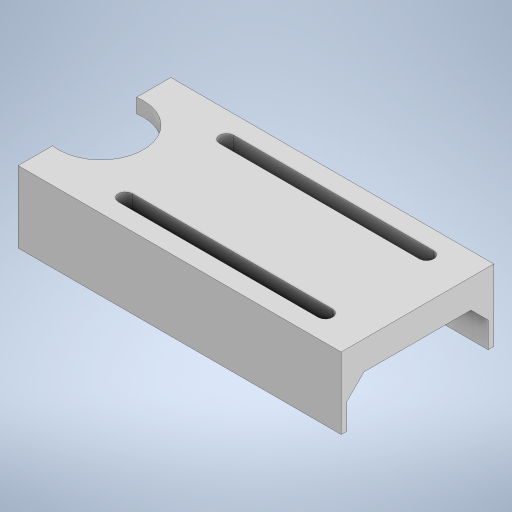
# Autodesk Inventor part: klapa
Saved by Autodesk Inventor 2024.3 (Build 283343000, 343)
## iProperties
Created: 2024-08-09
Part Number: klapa
Material: Ogólny
Document SubType Name: Modeling
Designer: User
Density: 1 g/cm^3
Appearance: Domyślna
Author: User
Autodesk Inventor part; units mm, degrees
ref_plane "YZ Plane" through (0, 0, 0) normal (1, 0, 0) x (0, 1, 0)
ref_plane "XZ Plane" through (0, 0, 0) normal (0, 1, 0) x (-1, 0, 0)
ref_plane "XY Plane" through (0, 0, 0) normal (0, 0, 1) x (1, 0, 0)
sketch "Szkic1" plane through (0, 0, 0) normal (0, 1, 0) x (-1, 0, 0)
  line L0 (0, 0) -> (0, -49.4)
  line L1 (0, 0) -> (108, 0)
  line L2 (0, 0) -> (108.995, 0)
  line L3 (108.995, 0) -> (108.995, -49.4)
  line L4 (108.995, -49.4) -> (0, -49.4)
  line L5 (0, -49.4) -> (0, 0)
  line L6 (0, 0) -> (0, 2)
  line L7 (0, 2) -> (-2, 2)
  line L8 (108.995, -49.4) -> (110.995, -49.4)
  line L9 (110.995, -49.4) -> (110.995, -51.4)
  line L10 (110.995, -51.4) -> (-2, -51.4)
  line L11 (-2, -51.4) -> (-2, 2)
  line L12 (-2, 2) -> (110.995, 2)
  line L13 (110.995, 2) -> (110.995, -51.4)
  line L14 (110.995, 2) -> (100.995, 2)
  line L15 (100.995, 2) -> (100.995, 0)
  line L16 (110.995, -51.4) -> (100.995, -51.4)
  line L17 (100.995, -51.4) -> (100.995, -49.4)
  line L18 (-2, 2) -> (8, 2)
  line L19 (8, 2) -> (8, 0)
  line L20 (-2, -51.4) -> (8, -51.4)
  line L21 (8, -51.4) -> (8, -49.4)
  line L22 (-2, 0) -> (0, 0)
  line L23 (108.995, 0) -> (110.995, 0)
  line L24 (108.995, -49.4) -> (110.995, -49.4)
  line L25 (-2, -49.4) -> (0, -49.4)
  line L26 (100.995, 2) -> (90.995, 2)
  line L27 (90.995, 2) -> (90.995, 0)
  line L28 (100.995, -51.4) -> (90.995, -51.4)
  line L29 (90.995, -51.4) -> (90.995, -49.4)
  line L30 (110.995, -24.7) -> (-2, -24.7)
  line L31 (54.4975, -51.4) -> (54.4975, 2)
  line L32 (90.995, 2) -> (60.995, 2)
  line L33 (60.995, 2) -> (60.995, 0)
  line L34 (48, 2) -> (48, 0)
  line L35 (60.995, -51.4) -> (60.995, -49.4)
  line L36 (48, -51.4) -> (48, -49.4)
  point P0 (48, 0)
  dimension "d0" = 49.4
  dimension "d1" = 108
  dimension "d2" = 2
  dimension "d3" = 2
  dimension "d4" = 2
  dimension "d5" = 2
  dimension "d6" = 10
  dimension "d7" = 10
  dimension "d8" = 10
  dimension "d9" = 10
  dimension "d16" = 10
  dimension "d17" = 10
  dimension "d33" = 30
  constraints: 74 end point, 20 point on line, 12 perpendicular, 6 symmetric about line, 5 parallel, 4 horizontal, 4 midpoint, 2 vertical
  measures "d0" distance of L0.start L0.end
  measures "d1" distance of L0.start L1.end
  measures "d2" distance of L0.start L6.end
  measures "d3" distance of L6.end L7.end
  measures "d4" distance of L3.end L8.end
  measures "d5" distance of L8.end L9.end
  measures "d6" distance of L12.end L14.end
  measures "d7" distance of L9.end L16.end
  measures "d8" distance of L7.end L18.end
  measures "d9" distance of L10.end L20.end
  measures "d16" distance of L14.end L26.end
  measures "d17" distance of L16.end L28.end
  measures "d33" distance of L26.end L32.end
extrude "Wyciągnięcie proste1" add sketch "Szkic1" along normal blind 20 contours L6 L12 L19 L1 | L22 L11 L7 L6 | L19 L12 L34 L1 | L4 L21 L10 L11 L25 | L34 L12 L31 L1 | L4 L36 L10 L21 | L31 L10 L36 L4 | L4 L35 L10 L31 | L31 L12 L33 L1 | L2 L1 L15 L12 L13 L23 | L8 L9 L10 L17 L4 | L4 L29 L10 L35 | L33 L12 L27 L1 | L17 L10 L29 L4 | L27 L12 L15 L1
sketch "Szkic2" plane through (0, 20, 0) normal (0, 1, 0) x (1, 0, 0)
  line L0 (-8, -2) -> (2, -2) projected
  line L1 (2, 51.4) -> (-110.995, 51.4) projected
  line L2 (2, -2) -> (-110.995, -2)
  line L3 (-110.995, -2) -> (-110.995, 51.4)
  line L4 (-110.995, 51.4) -> (2, 51.4)
  line L5 (2, 51.4) -> (2, -2)
  line L6 (-110.995, 0) -> (-110.995, 10)
  line L7 (-110.995, 49.4) -> (2, 49.4) projected
  line L8 (-110.995, 49.4) -> (-110.995, 39.4)
  arc A0 (-110.995, 10) -> (-110.995, 39.4) centre (-125.3914, 24.7) ccw
  arc A1 (-110.995, 10) -> (-110.995, 39.4) centre (-108.7482, 24.7) ccw
  point P0 (0, 0)
  point P1 (-100.995, 51.4)
  point P2 (-100.995, 49.4)
  point P3 (-100.995, 51.4)
  point P4 (-90.995, 51.4)
  point P5 (-90.995, 49.4)
  point P6 (-60.995, 51.4)
  point P7 (-60.995, 49.4)
  dimension "d12" = 10
  dimension "d13" = 10
  constraints: 12 end point, 4 point on circle, 3 point on line, 2 centre point, 2 parallel, 1 horizontal, 1 perpendicular
  measures "d12" distance of L6.start L6.end
  measures "d13" distance of L7.start L8.end
extrude "Wyciągnięcie proste2" add sketch "Szkic2" along normal blind 5 contours L2 L3 A1 L7 L5 L0 | L7 L3 L1 L5
sketch "Szkic3" plane through (2, 0, -49.4) normal (1, 0, 0) x (0, 0, -1)
  line L0 (-39.4, 25) -> (-51.4, 25) projected
  line L1 (2, 0) -> (2, 20) projected
  line L2 (-51.4, 25) -> (2, 25)
  line L3 (2, 25) -> (2, 15)
  line L4 (2, 15) -> (-51.4, 15)
  line L5 (-51.4, 15) -> (-51.4, 25)
  point P0 (-49.4, 0)
  dimension "d18" = 10
  constraints: 8 end point, 2 parallel, 1 horizontal, 1 perpendicular, 1 point on line
  measures "d18" distance of L2.end L3.end
extrude "Wyciągnięcie proste3" add sketch "Szkic3" against normal blind 1
chamfer "Faza1" distance 6 angle 45 2 edges at (1.5, 15, 0) (1.5, 15, -49.4)
sketch "Szkic5" plane through (0, 25, 0) normal (0, 1, 0) x (1, 0, 0)
  line L0 (-110.995, -2) -> (2, -2) projected
  line L1 (2, -2) -> (2, 7)
  line L2 (2, -2) -> (11, -2) construction
  line L3 (2, 7) -> (-12.5, 7)
  line L4 (-54.4975, -2) -> (-54.4975, 51.4)
  line L5 (2, 51.4) -> (-110.995, 51.4) projected
  line L6 (2, -2) -> (2, 51.4) projected
  line L7 (2, 24.7) -> (-94.0806, 24.7)
  line L8 (-110.995, 7) -> (-96.495, 7)
  line L9 (2, 42.4) -> (-12.5, 42.4)
  line L10 (-110.995, 42.4) -> (-96.495, 42.4)
  line L11 (-12.5, 7) -> (-82.5, 7) construction
  line L12 (-12.5, 9.5) -> (-82.5, 9.5)
  line L13 (-82.5, 4.5) -> (-12.5, 4.5)
  arc A0 (-12.5, 4.5) -> (-12.5, 9.5) centre (-12.5, 7) ccw
  arc A1 (-82.5, 9.5) -> (-82.5, 4.5) centre (-82.5, 7) ccw
  line L14 (-12.5, 42.4) -> (-82.5, 42.4) construction
  line L15 (-12.5, 44.9) -> (-82.5, 44.9)
  line L16 (-82.5, 39.9) -> (-12.5, 39.9)
  arc A2 (-12.5, 39.9) -> (-12.5, 44.9) centre (-12.5, 42.4) ccw
  arc A3 (-82.5, 44.9) -> (-82.5, 39.9) centre (-82.5, 42.4) ccw
  line L17 (-12.5, 42.4) -> (57.5, 42.4) construction
  point P0 (0, 0)
  point P1 (-47.5, 7)
  point P2 (-47.5, 42.4)
  dimension "d37" = 9
  dimension "d38" = 90
  dimension "d39" = 14.5
  dimension "d40" = 70
  dimension "d41" = 5
  dimension "d42" = 70
  dimension "d43" = 180
  dimension "d44" = 5
  constraints: 34 end point, 8 point on circle, 8 tangent, 6 symmetric about line, 5 midpoint, 4 centre point, 4 horizontal, 2 equal length, 2 parallel, 1 collinear, 1 point on line, 1 vertical
  measures "d37" distance of L0.end L1.end
  measures "d38" angle of L2 L1
  measures "d39" distance of L1.end L3.end
  measures "d40" distance of L3.end L11.end
  measures "d41" diameter of A1
  measures "d42" distance of L9.end L14.end
  measures "d43" angle of L14 L17
  measures "d44" diameter of A3
extrude "Wyciągnięcie proste5" cut sketch "Szkic5" against normal blind 20 contours L13 A1 L12 L4 | L4 L12 A0 L13 | L16 A3 L15 L4 | L4 L15 A2 L16
